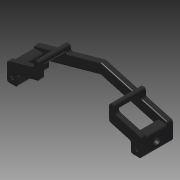
# Autodesk Inventor part: Solenoid Mount
Saved by Autodesk Inventor 2015 (Build 190159000, 159)
## iProperties
Created: 2016-09-23
Part Number: Solenoid Mount
Material: Generic
Document SubType Name: Modeling
Designer: James Yelland
Density: 1 g/cm^3
Appearance: Default
Author: James Yelland
Autodesk Inventor part; units mm, degrees
ref_plane "YZ Plane" through (0, 0, 0) normal (1, 0, 0) x (0, 1, 0)
ref_plane "XZ Plane" through (0, 0, 0) normal (0, 1, 0) x (-1, 0, 0)
ref_plane "XY Plane" through (0, 0, 0) normal (0, 0, 1) x (1, 0, 0)
sketch "Sketch1" plane through (0, 0, 0) normal (0, 1, 0) x (-1, 0, 0)
  line L0 (-54.007353, -78) -> (-54.007353, -71.520227)
  arc A0 (-52.542573, -69.593172) -> (-54.007353, -71.520227) centre (-52.007353, -71.520227) ccw
  arc A1 (-56.007353, -80) -> (-54.007353, -78) centre (-56.007353, -78) ccw
  line L1 (-54.007353, -78) -> (-54.007353, -71.520227)
  arc A2 (-52.542573, -69.593172) -> (-54.007353, -71.520227) centre (-52.007353, -71.520227) ccw
  arc A3 (-56.007353, -80) -> (-54.007353, -78) centre (-56.007353, -78) ccw
  line L2 (-54.007353, -78) -> (-54.007353, -71.520227)
  arc A4 (-52.542573, -69.593172) -> (-54.007353, -71.520227) centre (-52.007353, -71.520227) ccw
  arc A5 (-56.007353, -80) -> (-54.007353, -78) centre (-56.007353, -78) ccw
  line L3 (-62.007353, -80) -> (-56.007353, -80)
  line L4 (-64.007353, -78) -> (-64.007353, -64.297626)
  arc A6 (-62.542573, -62.370572) -> (-64.007353, -64.297626) centre (-62.007353, -64.297626) ccw
  arc A7 (-64.007353, -78) -> (-62.007353, -80) centre (-62.007353, -78) ccw
  line L5 (-52.542573, -69.593172) -> (-34.736806, -64.647799)
  line L6 (-33.272027, -62.720745) -> (-33.272027, -56.33805)
  line L7 (-33.272027, -56.33805) -> (-33.272027, -54)
  line L8 (-33.272027, -54) -> (-33.272027, -51)
  line L9 (-35.272027, -49) -> (-36.272027, -49)
  line L10 (-62.542573, -62.370572) -> (-39.736806, -56.036499)
  line L11 (-38.272027, -54.109444) -> (-38.272027, -51)
  arc A8 (-36.272027, -49) -> (-38.272027, -51) centre (-36.272027, -51) ccw
  arc A9 (-33.272027, -51) -> (-35.272027, -49) centre (-35.272027, -51) ccw
  arc A10 (-39.736806, -56.036499) -> (-38.272027, -54.109444) centre (-40.272027, -54.109444) ccw
  arc A11 (-34.736806, -64.647799) -> (-33.272027, -62.720745) centre (-35.272027, -62.720745) ccw
  line L12 (54.007353, -78) -> (54.007353, -71.520227)
  arc A12 (54.007353, -71.520227) -> (52.542573, -69.593172) centre (52.007353, -71.520227) ccw
  arc A13 (54.007353, -78) -> (56.007353, -80) centre (56.007353, -78) ccw
  line L13 (54.007353, -78) -> (54.007353, -71.520227)
  arc A14 (54.007353, -71.520227) -> (52.542573, -69.593172) centre (52.007353, -71.520227) ccw
  arc A15 (54.007353, -78) -> (56.007353, -80) centre (56.007353, -78) ccw
  line L14 (54.007353, -78) -> (54.007353, -71.520227)
  arc A16 (54.007353, -78) -> (56.007353, -80) centre (56.007353, -78) ccw
  arc A17 (54.007353, -71.520227) -> (52.542573, -69.593172) centre (52.007353, -71.520227) ccw
  line L15 (62.007353, -80) -> (56.007353, -80)
  line L16 (64.007353, -78) -> (64.007353, -64.297626)
  arc A18 (64.007353, -64.297626) -> (62.542573, -62.370572) centre (62.007353, -64.297626) ccw
  arc A19 (62.007353, -80) -> (64.007353, -78) centre (62.007353, -78) ccw
  line L17 (52.542573, -69.593172) -> (34.736806, -64.647799)
  line L18 (33.272027, -62.720745) -> (33.272027, -56.33805)
  line L19 (33.272027, -56.33805) -> (33.272027, -54)
  line L20 (33.272027, -54) -> (33.272027, -51)
  line L21 (35.272027, -49) -> (36.272027, -49)
  line L22 (62.542573, -62.370572) -> (39.736806, -56.036499)
  line L23 (38.272027, -54.109444) -> (38.272027, -51)
  arc A20 (38.272027, -51) -> (36.272027, -49) centre (36.272027, -51) ccw
  arc A21 (35.272027, -49) -> (33.272027, -51) centre (35.272027, -51) ccw
  arc A22 (38.272027, -54.109444) -> (39.736806, -56.036499) centre (40.272027, -54.109444) ccw
  arc A23 (33.272027, -62.720745) -> (34.736806, -64.647799) centre (35.272027, -62.720745) ccw
  point P0 (-33.272027, -64.240971)
  point P1 (-33.272027, -49)
  point P2 (-38.272027, -49)
  point P3 (33.272027, -64.240971)
  point P4 (33.272027, -49)
  point P5 (38.272027, -49)
  dimension "d11" = 2
  dimension "d29" = 20
  dimension "d30" = 5
  dimension "d31" = 5
  dimension "d32" = 2
  constraints: 48 end point, 48 point on circle, 24 centre point, 16 point on line, 13 tangent, 4 equal radius, 2 perpendicular, 1 vertical
  measures "d11" radius of A6
  measures "d29" distance of L5.start point (-33.272, -64.241)
  measures "d30" distance of L7.end point (-33.272, -49)
  measures "d31" distance of point (-33.272, -49) point (-38.272, -49)
  measures "d32" radius of A8
extrude "Extrusion1" add sketch "Sketch1" along normal blind 5
sketch "Sketch2" plane through (0, 5, 0) normal (0, 1, 0) x (1, 0, 0)
  line L0 (54.007353, 78) -> (54.007353, 71.520227)
  arc A0 (56.007353, 80) -> (54.007353, 78) centre (56.007353, 78) ccw
  line L1 (62.007353, 80) -> (56.007353, 80)
  arc A1 (64.007353, 78) -> (62.007353, 80) centre (62.007353, 78) ccw
  line L2 (64.007353, 64.297626) -> (64.007353, 78)
  line L3 (54.007353, 71.520227) -> (54.007353, 66.297626)
  line L4 (56.007353, 64.297626) -> (62.007353, 64.297626)
  line L5 (64.007353, 66.297626) -> (64.007353, 78)
  arc A2 (62.007353, 64.297626) -> (64.007353, 66.297626) centre (62.007353, 66.297626) ccw
  arc A3 (54.007353, 66.297626) -> (56.007353, 64.297626) centre (56.007353, 66.297626) ccw
  line L6 (0, 44.070657) -> (0, 74.760113)
  line L7 (-54.007353, 78) -> (-54.007353, 71.520227)
  arc A4 (-54.007353, 78) -> (-56.007353, 80) centre (-56.007353, 78) ccw
  line L8 (-62.007353, 80) -> (-56.007353, 80)
  arc A5 (-62.007353, 80) -> (-64.007353, 78) centre (-62.007353, 78) ccw
  line L9 (-64.007353, 64.297626) -> (-64.007353, 78)
  line L10 (-54.007353, 71.520227) -> (-54.007353, 66.297626)
  line L11 (-56.007353, 64.297626) -> (-62.007353, 64.297626)
  line L12 (-64.007353, 66.297626) -> (-64.007353, 78)
  arc A6 (-64.007353, 66.297626) -> (-62.007353, 64.297626) centre (-62.007353, 66.297626) ccw
  arc A7 (-56.007353, 64.297626) -> (-54.007353, 66.297626) centre (-56.007353, 66.297626) ccw
  line L13 (38.272027, 51) -> (38.272027, 54.109444)
  arc A8 (36.272027, 49) -> (38.272027, 51) centre (36.272027, 51) ccw
  line L14 (35.272027, 49) -> (36.272027, 49)
  arc A9 (33.272027, 51) -> (35.272027, 49) centre (35.272027, 51) ccw
  line L15 (33.272027, 62.720745) -> (33.272027, 51)
  line L16 (36.272027, 49) -> (35.272027, 49)
  line L17 (35.772027, 49) -> (35.772027, 54)
  line L18 (35.772027, 54) -> (35.272027, 54)
  line L19 (33.272027, 51) -> (33.272027, 62.720745)
  line L20 (35.772027, 54) -> (36.272027, 54)
  line L21 (38.272027, 54.109444) -> (38.272027, 51)
  line L22 (-38.272027, 51) -> (-38.272027, 52)
  arc A10 (-38.272027, 51) -> (-36.272027, 49) centre (-36.272027, 51) ccw
  line L23 (-35.272027, 49) -> (-36.272027, 49)
  arc A11 (-35.272027, 49) -> (-33.272027, 51) centre (-35.272027, 51) ccw
  line L24 (-33.272027, 52) -> (-33.272027, 51)
  line L25 (-36.272027, 49) -> (-35.272027, 49)
  line L26 (-35.772027, 49) -> (-35.772027, 54)
  line L27 (-35.772027, 54) -> (-35.272027, 54)
  line L28 (-33.272027, 51) -> (-33.272027, 62.720745)
  line L29 (-35.772027, 54) -> (-36.272027, 54)
  line L30 (-38.272027, 54.109444) -> (-38.272027, 51)
  line L31 (38.272027, 52) -> (38.272027, 51)
  line L32 (33.272027, 52) -> (33.272027, 51)
  arc A12 (-33.272027, 52) -> (-35.272027, 54) centre (-35.272027, 52) ccw
  arc A13 (-36.272027, 54) -> (-38.272027, 52) centre (-36.272027, 52) ccw
  arc A14 (38.272027, 52) -> (36.272027, 54) centre (36.272027, 52) ccw
  arc A15 (35.272027, 54) -> (33.272027, 52) centre (35.272027, 52) ccw
  point P0 (0, 0)
  point P1 (33.272027, 54)
  point P2 (38.272027, 54)
  point P3 (-33.272027, 54)
  point P4 (-38.272027, 54)
  dimension "d19" = 2
  dimension "d33" = 5
  dimension "d34" = 2
  constraints: 48 end point, 26 symmetric about line, 24 point on circle, 16 point on line, 12 centre point, 12 tangent, 4 equal radius, 4 vertical, 2 collinear, 2 perpendicular, 1 horizontal, 1 midpoint, 6 other
  measures "d19" radius of A2
  measures "d33" distance of L17.start L17.end
  measures "d34" radius of A12
extrude "Extrusion2" add sketch "Sketch2" along normal blind 20
sketch "Sketch3" plane through (0, 25, 0) normal (0, 1, 0) x (1, 0, 0)
  arc A0 (62.007353, 64.297626) -> (64.007353, 66.297626) centre (62.007353, 66.297626) ccw
  line L0 (62.007353, 64.297626) -> (56.007353, 64.297626)
  arc A1 (54.007353, 66.297626) -> (56.007353, 64.297626) centre (56.007353, 66.297626) ccw
  line L1 (54.007353, 66.297626) -> (54.007353, 71.520227)
  arc A2 (52.542573, 69.593172) -> (54.007353, 71.520227) centre (52.007353, 71.520227) ccw
  line L2 (52.542573, 69.593172) -> (34.736806, 64.647799)
  arc A3 (34.736806, 64.647799) -> (33.272027, 62.720745) centre (35.272027, 62.720745) ccw
  line L3 (33.272027, 62.720745) -> (33.272027, 52)
  arc A4 (35.272027, 54) -> (33.272027, 52) centre (35.272027, 52) ccw
  line L4 (35.272027, 54) -> (36.272027, 54)
  arc A5 (38.272027, 52) -> (36.272027, 54) centre (36.272027, 52) ccw
  line L5 (38.272027, 52) -> (38.272027, 54.109444)
  arc A6 (39.736806, 56.036499) -> (38.272027, 54.109444) centre (40.272027, 54.109444) ccw
  line L6 (39.736806, 56.036499) -> (62.542573, 62.370572)
  arc A7 (62.542573, 62.370572) -> (64.007353, 64.297626) centre (62.007353, 64.297626) ccw
  line L7 (64.007353, 64.297626) -> (64.007353, 66.297626)
  line L8 (54.007353, 78) -> (54.007353, 66.297626)
  arc A8 (54.007353, 66.297626) -> (56.007353, 64.297626) centre (56.007353, 66.297626) ccw
  line L9 (56.007353, 64.297626) -> (62.007353, 64.297626)
  arc A9 (62.007353, 64.297626) -> (64.007353, 66.297626) centre (62.007353, 66.297626) ccw
  line L10 (64.007353, 66.297626) -> (64.007353, 78)
  arc A10 (64.007353, 78) -> (62.007353, 80) centre (62.007353, 78) ccw
  line L11 (62.007353, 80) -> (56.007353, 80)
  arc A11 (56.007353, 80) -> (54.007353, 78) centre (56.007353, 78) ccw
  line L12 (38.272027, 51) -> (38.272027, 52)
  arc A12 (38.272027, 52) -> (36.272027, 54) centre (36.272027, 52) ccw
  line L13 (36.272027, 54) -> (35.272027, 54)
  arc A13 (35.272027, 54) -> (33.272027, 52) centre (35.272027, 52) ccw
  line L14 (33.272027, 52) -> (33.272027, 51)
  arc A14 (33.272027, 51) -> (35.272027, 49) centre (35.272027, 51) ccw
  line L15 (35.272027, 49) -> (36.272027, 49)
  arc A15 (36.272027, 49) -> (38.272027, 51) centre (36.272027, 51) ccw
  arc A16 (-33.272027, 52) -> (-35.272027, 54) centre (-35.272027, 52) ccw
  line L16 (-33.272027, 52) -> (-33.272027, 62.720745)
  arc A17 (-33.272027, 62.720745) -> (-34.736806, 64.647799) centre (-35.272027, 62.720745) ccw
  line L17 (-34.736806, 64.647799) -> (-52.542573, 69.593172)
  arc A18 (-54.007353, 71.520227) -> (-52.542573, 69.593172) centre (-52.007353, 71.520227) ccw
  line L18 (-54.007353, 71.520227) -> (-54.007353, 66.297626)
  arc A19 (-56.007353, 64.297626) -> (-54.007353, 66.297626) centre (-56.007353, 66.297626) ccw
  line L19 (-56.007353, 64.297626) -> (-62.007353, 64.297626)
  arc A20 (-64.007353, 66.297626) -> (-62.007353, 64.297626) centre (-62.007353, 66.297626) ccw
  line L20 (-64.007353, 66.297626) -> (-64.007353, 64.297626)
  arc A21 (-64.007353, 64.297626) -> (-62.542573, 62.370572) centre (-62.007353, 64.297626) ccw
  line L21 (-62.542573, 62.370572) -> (-39.736806, 56.036499)
  arc A22 (-38.272027, 54.109444) -> (-39.736806, 56.036499) centre (-40.272027, 54.109444) ccw
  line L22 (-38.272027, 54.109444) -> (-38.272027, 52)
  arc A23 (-36.272027, 54) -> (-38.272027, 52) centre (-36.272027, 52) ccw
  line L23 (-36.272027, 54) -> (-35.272027, 54)
  line L24 (-36.272027, 49) -> (-35.272027, 49)
  arc A24 (-35.272027, 49) -> (-33.272027, 51) centre (-35.272027, 51) ccw
  line L25 (-33.272027, 51) -> (-33.272027, 52)
  arc A25 (-33.272027, 52) -> (-35.272027, 54) centre (-35.272027, 52) ccw
  line L26 (-35.272027, 54) -> (-36.272027, 54)
  arc A26 (-36.272027, 54) -> (-38.272027, 52) centre (-36.272027, 52) ccw
  line L27 (-38.272027, 52) -> (-38.272027, 51)
  arc A27 (-38.272027, 51) -> (-36.272027, 49) centre (-36.272027, 51) ccw
  line L28 (-54.007353, 66.297626) -> (-54.007353, 78)
  arc A28 (-54.007353, 78) -> (-56.007353, 80) centre (-56.007353, 78) ccw
  line L29 (-56.007353, 80) -> (-62.007353, 80)
  arc A29 (-62.007353, 80) -> (-64.007353, 78) centre (-62.007353, 78) ccw
  line L30 (-64.007353, 78) -> (-64.007353, 66.297626)
  arc A30 (-64.007353, 66.297626) -> (-62.007353, 64.297626) centre (-62.007353, 66.297626) ccw
  line L31 (-62.007353, 64.297626) -> (-56.007353, 64.297626)
  arc A31 (-56.007353, 64.297626) -> (-54.007353, 66.297626) centre (-56.007353, 66.297626) ccw
  line L32 (52.542573, 69.593172) -> (0.53522, 55.148652)
  line L33 (34.736806, 64.647799) -> (52.542573, 69.593172)
  line L34 (-0.53522, 55.148652) -> (-34.736806, 64.647799)
  line L35 (0.53522, 45.148652) -> (30.736806, 53.536839)
  line L36 (-0.53522, 45.148652) -> (-30.736806, 53.536839)
  arc A32 (-0.53522, 45.148652) -> (0.53522, 45.148652) centre (0, 47.075707) ccw
  arc A33 (-0.53522, 55.148652) -> (0.53522, 55.148652) centre (0, 57.075707) ccw
  line L37 (33.272027, 51) -> (33.272027, 62.720745)
  line L38 (33.272027, 51.609785) -> (33.272027, 51)
  arc A34 (33.272027, 51.609785) -> (30.736806, 53.536839) centre (31.272027, 51.609785) ccw
  line L39 (-33.272027, 51) -> (-33.272027, 51.609785)
  line L40 (-33.272027, 52) -> (-33.272027, 62.720745)
  arc A35 (-30.736806, 53.536839) -> (-33.272027, 51.609785) centre (-31.272027, 51.609785) ccw
  line L41 (-34.736806, 64.647799) -> (-52.542573, 69.593172)
  arc A36 (-54.007353, 71.520227) -> (-52.542573, 69.593172) centre (-52.007353, 71.520227) ccw
  arc A37 (-54.007353, 71.520227) -> (-52.542573, 69.593172) centre (-52.007353, 71.520227) ccw
  arc A38 (-54.007353, 78) -> (-56.007353, 80) centre (-56.007353, 78) ccw
  arc A39 (-62.007353, 80) -> (-64.007353, 78) centre (-62.007353, 78) ccw
  arc A40 (-64.007353, 64.297626) -> (-62.542573, 62.370572) centre (-62.007353, 64.297626) ccw
  arc A41 (-38.272027, 54.109444) -> (-39.736806, 56.036499) centre (-40.272027, 54.109444) ccw
  arc A42 (-38.272027, 51) -> (-36.272027, 49) centre (-36.272027, 51) ccw
  arc A43 (-35.272027, 49) -> (-33.272027, 51) centre (-35.272027, 51) ccw
  arc A44 (52.542573, 69.593172) -> (54.007353, 71.520227) centre (52.007353, 71.520227) ccw
  arc A45 (56.007353, 80) -> (54.007353, 78) centre (56.007353, 78) ccw
  arc A46 (64.007353, 78) -> (62.007353, 80) centre (62.007353, 78) ccw
  arc A47 (62.542573, 62.370572) -> (64.007353, 64.297626) centre (62.007353, 64.297626) ccw
  arc A48 (39.736806, 56.036499) -> (38.272027, 54.109444) centre (40.272027, 54.109444) ccw
  arc A49 (36.272027, 49) -> (38.272027, 51) centre (36.272027, 51) ccw
  arc A50 (33.272027, 51) -> (35.272027, 49) centre (35.272027, 51) ccw
  line L42 (38.272027, 54.109444) -> (38.272027, 51)
  line L43 (36.272027, 49) -> (35.272027, 49)
  line L44 (39.736806, 56.036499) -> (62.542573, 62.370572)
  line L45 (64.007353, 64.297626) -> (64.007353, 78)
  line L46 (62.007353, 80) -> (56.007353, 80)
  line L47 (54.007353, 78) -> (54.007353, 71.520227)
  arc A51 (52.542573, 69.593172) -> (54.007353, 71.520227) centre (52.007353, 71.520227) ccw
  arc A52 (56.007353, 80) -> (54.007353, 78) centre (56.007353, 78) ccw
  line L48 (-54.007353, 71.520227) -> (-54.007353, 78)
  arc A53 (-54.007353, 78) -> (-56.007353, 80) centre (-56.007353, 78) ccw
  line L49 (-56.007353, 80) -> (-62.007353, 80)
  line L50 (-62.007353, 80) -> (-56.007353, 80)
  line L51 (-64.007353, 78) -> (-64.007353, 64.297626)
  line L52 (-62.542573, 62.370572) -> (-39.736806, 56.036499)
  line L53 (-62.542573, 62.370572) -> (-39.736806, 56.036499)
  line L54 (-38.272027, 54.109444) -> (-38.272027, 51)
  line L55 (-36.272027, 49) -> (-35.272027, 49)
  arc A54 (-38.272027, 51) -> (-36.272027, 49) centre (-36.272027, 51) ccw
  point P0 (0, 0)
  point P1 (33.272027, 54.240971)
  point P2 (-33.272027, 54.240971)
  dimension "d61" = 2
  dimension "d62" = 2
  dimension "d63" = 2
  dimension "d64" = 2
  constraints: 38 end point, 36 point on circle, 18 centre point, 14 coincident, 13 tangent, 8 point on line, 7 collinear, 6 vertical, 2 horizontal
  measures "d61" radius of A32
  measures "d62" radius of A33
  measures "d63" radius of A34
  measures "d64" radius of A35
extrude "Extrusion3" add sketch "Sketch3" along normal blind 5
sketch "Sketch4" plane through (0, 30, 0) normal (0, 1, 0) x (1, 0, 0)
  line L0 (54.007353, 71.520227) -> (54.007353, 78)
  line L1 (54.007353, 74.760113) -> (59.247353, 74.760113)
  circle A0 centre (59.247353, 74.760113) radius 1.6
  line L2 (-54.007353, 78) -> (-54.007353, 71.520227)
  line L3 (-54.007353, 74.760113) -> (-59.247353, 74.760113)
  circle A1 centre (-59.247353, 74.760113) radius 1.6
  point P0 (0, 0)
  dimension "d37" = 5.24
  dimension "d38" = 3.2
  dimension "d39" = 5.24
  dimension "d40" = 3.2
  constraints: 4 end point, 2 centre point, 2 coincident, 2 horizontal, 2 midpoint
  measures "d37" distance of L1.start L1.end
  measures "d38" diameter of A0
  measures "d39" distance of L3.start L3.end
  measures "d40" diameter of A1
extrude "Extrusion4" cut sketch "Sketch4" against normal through all
fillet "Fillet1" radius 1 18 edges at (63.5996, 5, -63.0873) (64.0074, 5, -65.2976) (38.6798, 5, -55.3197) (38.272, 5, -53.0547) (51.1397, 5, -59.2035) (33.272, 5, -57.3604) (43.6397, 5, -67.1205) (53.5996, 5, -70.3099) (33.6798, 5, -63.931) (-53.5996, 5, -70.3099) (-33.6798, 5, -63.931) (-33.272, 5, -57.3604) (-43.6397, 5, -67.1205) (-38.272, 5, -53.0547) (-51.1397, 5, -59.2035) (-63.5996, 5, -63.0873) (-64.0074, 5, -65.2976) (-38.6798, 5, -55.3197)
fillet "Fillet2" radius 1 10 edges at (53.5996, 25, -70.3099) (64.0074, 25, -65.2976) (51.1397, 25, -59.2035) (-26.5389, 25, -62.3709) (-53.5996, 25, -70.3099) (-38.6798, 25, -55.3197) (-38.272, 25, -53.0547) (-63.5996, 25, -63.0873) (-64.0074, 25, -65.2976) (-51.1397, 25, -59.2035)
sketch "Sketch5" plane through (54.007353, 0, -78) normal (-1, 0, 0) x (0, 0, 1)
  line L0 (0, 30) -> (6.479773, 30)
  line L1 (6.479773, 30) -> (5.479773, 30)
  line L2 (5.479773, 30) -> (5.479773, 15)
  circle A0 centre (5.479773, 15) radius 3.25
  point P0 (78, 0)
  dimension "d48" = 1
  dimension "d49" = 15
  dimension "d50" = 6.5
  constraints: 4 end point, 1 centre point, 1 coincident, 1 perpendicular, 1 point on line
  measures "d48" distance of L0.end L1.end
  measures "d49" distance of L1.end L2.end
  measures "d50" diameter of A0
extrude "Extrusion5" cut sketch "Sketch5" against normal through all
sketch "Sketch6" plane through (54.007353, 0, -78) normal (-1, 0, 0) x (0, 0, 1)
  circle A0 centre (5.479773, 15) radius 3.25
  circle A1 centre (5.479773, 15) radius 5
  point P0 (78, 0)
  dimension "d53" = 10
  constraints: 1 centre point, 1 coincident
  measures "d53" diameter of A1
extrude "Extrusion6" add sketch "Sketch6" along normal blind 2
chamfer "Chamfer1" distance 0.75 distance2 2 1 edges at (52.0074, 15, -77.5202) measured on face at (52.0074, 15, -77.0202)
fillet "Fillet3" radius 1 5 edges at (0, 25, -45.0757) (15.636, 25, -49.3427) (32.4823, 25, -53.202) (-32.4823, 25, -53.202) (-15.636, 25, -49.3427)
sketch "Sketch7" plane through (-54.007353, 0, -71.520227) normal (1, 0, 0) x (0, 0, -1)
  circle A0 centre (1, 15) radius 3.25 projected
  circle A1 centre (1, 15) radius 3
  point P0 (-71.520227, 0)
  dimension "d66" = 6
  constraints: 1 centre point, 1 coincident
  measures "d66" diameter of A1
extrude "Extrusion7" cut sketch "Sketch7" against normal blind 8 contours A1
body "Solid1"
